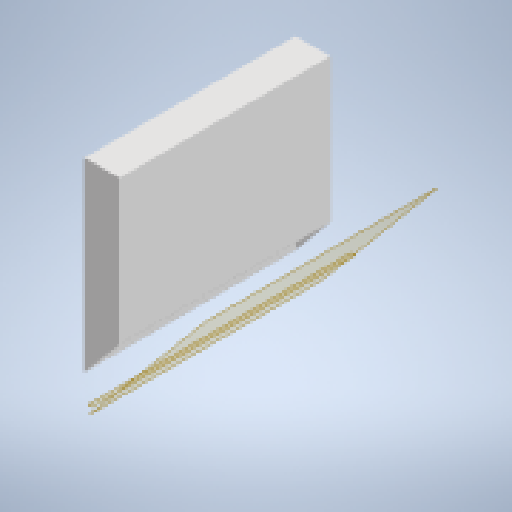
# Autodesk Inventor part: DUSTPAN
Saved by Autodesk Inventor 2024 (Build 280153000, 153)
## iProperties
Created: 2024-04-16
Part Number: DUSTPAN
Material: Generic
Document SubType Name: Modeling
Designer: teeta
Density: 1 g/cm^3
Appearance: Default
Author: teeta
Autodesk Inventor part; units mm, degrees
ref_plane "YZ Plane" through (0, 0, 0) normal (1, 0, 0) x (0, 1, 0)
ref_plane "XZ Plane" through (0, 0, 0) normal (0, 1, 0) x (-1, 0, 0)
ref_plane "XY Plane" through (0, 0, 0) normal (0, 0, 1) x (1, 0, 0)
ref_plane "Work Plane1" through (-12.7, 499.15, -25.4) normal (0, 1, 0) x (-1, 0, 0)
sketch "Sketch1" plane through (-12.7, 499.15, -25.4) normal (0, 1, 0) x (-1, 0, 0)
  line L0 (-19.05, 819.05) -> (-19.05, -19.05) projected
  line L1 (-12.7, 35.4) -> (-2.7, 35.4) projected
  line L2 (-12.7, 764.6) -> (-2.7, 764.6) projected
  line L3 (-19.05, 25.4) -> (105.4044, 25.4)
  line L4 (105.4044, 25.4) -> (105.4044, 774.6084)
  line L5 (105.4044, 774.6084) -> (-19.05, 774.6084)
  line L6 (-19.05, 774.6084) -> (-19.05, 25.4)
  point P0 (-12.7, 25.4)
  point P1 (-19.05, 774.6084)
  dimension "d0" = 749.2084
  dimension "d1" = 124.4544
  constraints: 8 end point, 2 parallel, 1 horizontal, 1 perpendicular, 1 point on line
  measures "d0" distance of L3.end L4.end
  measures "d1" distance of L4.end L5.end
extrude "Extrusion1" add sketch "Sketch1" along normal blind 661.25
ref_plane "Work Plane2" through (6.35, 499.15, 793.65) normal (0.7660444, -0.6427876, 0) x (0, 0, -1)
sketch "Sketch2" plane through (6.35, 499.15, 793.65) normal (0.7660444, -0.6427876, 0) x (0, 0, -1)
  line L0 (44.4416, 0) -> (44.4416, 506.5469) projected
  line L1 (44.4416, 167.8683) -> (793.65, 167.8683)
  line L2 (793.65, 167.8683) -> (793.65, -166.4116)
  line L3 (793.65, -166.4116) -> (44.4416, -166.4116)
  line L4 (44.4416, -166.4116) -> (44.4416, 167.8683)
  point P0 (793.65, -386.4528)
  constraints: 8 end point, 2 parallel, 1 horizontal, 1 perpendicular, 1 point on line
extrude "Extrusion2" cut sketch "Sketch2" against normal blind 96.5
shell "Shell1" thickness 5 removed faces 1 at (-35.1348, 599.8408, 499.4722)
body "Solid1"
